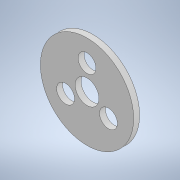
# Autodesk Inventor part: Rear Carrier
Saved by Autodesk Inventor 2022 (Build 260153000, 153)
## iProperties
Created: 2022-08-10
Part Number: Rear Carrier
Material: Generic
Document SubType Name: Modeling
Designer: Nick
Density: 1 g/cm^3
Appearance: Default
Author: Nick
Autodesk Inventor part; units mm, degrees
ref_plane "YZ Plane" through (0, 0, 0) normal (1, 0, 0) x (0, 1, 0)
ref_plane "XZ Plane" through (0, 0, 0) normal (0, 1, 0) x (-1, 0, 0)
ref_plane "XY Plane" through (0, 0, 0) normal (0, 0, 1) x (1, 0, 0)
sketch "Sketch1" plane through (0, 0, 0) normal (0, 0, 1) x (1, 0, 0)
  line L0 (0, 12.5) -> (10.8253, -6.25) construction
  line L1 (10.8253, -6.25) -> (-10.8253, -6.25) construction
  line L2 (-10.8253, -6.25) -> (0, 12.5) construction
  circle A0 centre (0, 0) radius 12.5 construction
  circle A1 centre (0, 12.5) radius 4.5
  circle A2 centre (-10.8253, -6.25) radius 4.5
  circle A3 centre (10.8253, -6.25) radius 4.5
  circle A4 centre (0, 0) radius 6
  circle A5 centre (0, 0) radius 23.495
  point P0 (-14.8427, -1.4622)
  point P1 (-6.1551, 13.5852)
  point P2 (6.1551, 13.5852)
  point P3 (9.5499, -13.0572)
  point P4 (-8.6876, -12.1231)
  dimension "d0" = 25
  dimension "d6" = 9
  dimension "d7" = 9
  dimension "d8" = 9
  dimension "d12" = 12
  dimension "d14" = 46.99
  constraints: 7 coincident, 6 end point, 5 centre point, 2 vertical alignment, 9 other
  measures "d6" diameter of A1
  measures "d7" diameter of A2
  measures "d8" diameter of A3
  measures "d12" diameter of A4
  measures "d14" diameter of A5
extrude "Extrusion1" add sketch "Sketch1" along normal blind 3 contours A1 | A2 | A3 | A4 | A5
extrude "Extrusion2" cut sketch "Sketch1" along normal through all contours A1 | A2 | A3 | A4
equation "\"d6\" = d7"
equation "\"d8\" = d7"
body "Solid1"
